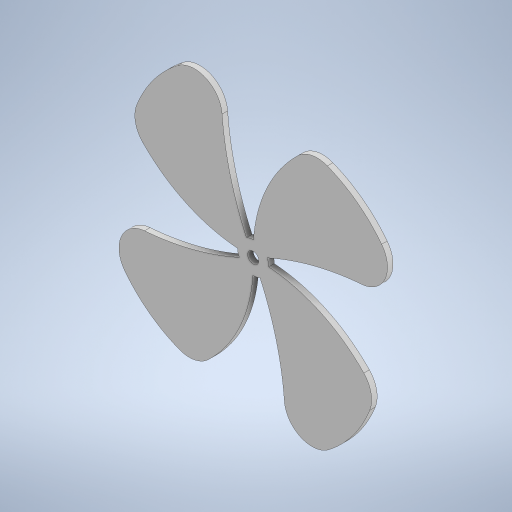
# Autodesk Inventor part: blades
Saved by Autodesk Inventor 2023.1 (Build 271208000, 208)
## iProperties
Created: 2023-05-29
Part Number: blades
Material: Generic
Document SubType Name: Modeling
Designer: Mansoor Lunawadi
Density: 1 g/cm^3
Appearance: Default
Author: Mansoor Lunawadi
Autodesk Inventor part; units mm, degrees
ref_plane "YZ Plane" through (0, 0, 0) normal (1, 0, 0) x (0, 1, 0)
ref_plane "XZ Plane" through (0, 0, 0) normal (0, 1, 0) x (-1, 0, 0)
ref_plane "XY Plane" through (0, 0, 0) normal (0, 0, 1) x (1, 0, 0)
sketch "Sketch1" plane through (0, 0, 0) normal (0, 0, 1) x (1, 0, 0)
  circle A0 centre (0, 0) radius 28
  circle A1 centre (0, 0) radius 1.8
  arc A2 (23.4652, 15.2769) -> (5.1796, 27.5168) centre (0, 0) ccw
  arc A3 (1.1742, 1.3642) -> (0.0115, 1.8) centre (0, 0) ccw
  arc A4 (1.3642, -1.1742) -> (1.8, -0.0115) centre (0, 0) ccw
  arc A5 (-1.3642, 1.1742) -> (-1.8, 0.0115) centre (0, 0) ccw
  arc A6 (-1.1742, -1.3642) -> (-0.0115, -1.8) centre (0, 0) ccw
  arc A7 (8.0598, 19.9487) -> (-0.0006, 1.8) centre (26.4682, 0.9087) ccw
  arc A8 (23.1644, 13.6701) -> (13.3624, 21.0083) centre (4.9305, -0.4702) ccw
  arc A9 (19.6092, 5.6217) -> (1.6116, 0.8017) centre (23.6763, -45.5755) ccw
  arc A10 (1.6116, 0.8017) -> (-0.0006, 1.8) centre (0, 0) ccw
  arc A11 (13.3624, 21.0083) -> (8.0598, 19.9487) centre (11.5352, 16.3541) ccw
  arc A12 (19.6092, 5.6217) -> (23.1644, 13.6701) centre (19.2133, 10.606) ccw
  arc A13 (19.9487, -8.0598) -> (1.8, 0.0006) centre (0.9087, -26.4682) ccw
  arc A14 (13.6701, -23.1644) -> (21.0083, -13.3624) centre (-0.4702, -4.9305) ccw
  arc A15 (5.6217, -19.6092) -> (0.8017, -1.6116) centre (-45.5755, -23.6763) ccw
  arc A16 (0.8017, -1.6116) -> (1.8, 0.0006) centre (0, 0) ccw
  arc A17 (21.0083, -13.3624) -> (19.9487, -8.0598) centre (16.3541, -11.5352) ccw
  arc A18 (5.6217, -19.6092) -> (13.6701, -23.1644) centre (10.606, -19.2133) ccw
  arc A19 (-1.1742, -1.3642) -> (-0.0115, -1.8) centre (0, 0) ccw
  arc A20 (-8.0598, -19.9487) -> (0.0006, -1.8) centre (-26.4682, -0.9087) ccw
  arc A21 (-23.1644, -13.6701) -> (-13.3624, -21.0083) centre (-4.9305, 0.4702) ccw
  arc A22 (-19.6092, -5.6217) -> (-23.1644, -13.6701) centre (-19.2133, -10.606) ccw
  arc A23 (-13.3624, -21.0083) -> (-8.0598, -19.9487) centre (-11.5352, -16.3541) ccw
  arc A24 (-19.6092, -5.6217) -> (-1.6116, -0.8017) centre (-23.6763, 45.5755) ccw
  arc A25 (-1.6116, -0.8017) -> (0.0006, -1.8) centre (0, 0) ccw
  arc A26 (-19.9487, 8.0598) -> (-1.8, -0.0006) centre (-0.9087, 26.4682) ccw
  arc A27 (-21.0083, 13.3624) -> (-19.9487, 8.0598) centre (-16.3541, 11.5352) ccw
  arc A28 (-5.6217, 19.6092) -> (-0.8017, 1.6116) centre (45.5755, 23.6763) ccw
  arc A29 (-13.6701, 23.1644) -> (-21.0083, 13.3624) centre (0.4702, 4.9305) ccw
  arc A30 (-5.6217, 19.6092) -> (-13.6701, 23.1644) centre (-10.606, 19.2133) ccw
  arc A31 (-0.8017, 1.6116) -> (-1.8, -0.0006) centre (0, 0) ccw
  circle A32 centre (0, 0) radius 1
  point P0 (0.0006, -1.8)
  point P1 (-1.6116, -0.8017)
  point P2 (-1.8, -0.0006)
  point P3 (-0.8017, 1.6116)
  point P4 (1.8, 0.0006)
  point P5 (0.8017, -1.6116)
  dimension "d2" = 5
  dimension "d3" = 5
  dimension "d4" = 5
  dimension "d5" = 5
  dimension "d6" = 5
  dimension "d7" = 5
  dimension "d8" = 5
  dimension "d9" = 5
  dimension "d15" = 3.6
  dimension "d16" = 2
  constraints: 65 point on circle, 33 centre point, 16 tangent, 4 coincident, 3 concentric
  measures "d2" radius of A11
  measures "d3" radius of A12
  measures "d4" radius of A17
  measures "d5" radius of A18
  measures "d6" radius of A23
  measures "d7" radius of A22
  measures "d8" radius of A27
  measures "d9" radius of A30
  measures "d15" diameter of A1
  measures "d16" diameter of A32
extrude "Extrusion1" add sketch "Sketch1" along normal blind 1 contours A13 A17 A14 A18 A15 A1 | A1 A7 A11 A8 A12 A9 | A20 A23 A21 A22 A24 A1 | A1 A26 A27 A29 A30 A28
sketch "Sketch2" plane through (0, 0, 0) normal (1, 0, 0) x (0, 1, 0)
  line L0 (0.9994, 0) -> (2.7994, 0)
  line L1 (2.7994, 0) -> (2.7994, 1)
  line L2 (2.7994, 1) -> (0.9994, 1)
  line L3 (0.9994, 1) -> (0.9994, 0)
  line L4 (0, -0.2) -> (0, 1.2) projected
  point P0 (0, 0)
  dimension "d12" = 1.8
  dimension "d13" = 1
  constraints: 8 end point, 2 parallel, 1 horizontal, 1 perpendicular
  measures "d12" distance of L2.end L1.end
  measures "d13" distance of L1.end L0.end
revolve "Revolution1" add sketch "Sketch2" angle 360 about axis through (0, 0, -10) along (0, 0, 1)
body "Solid1"
